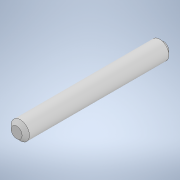
# Autodesk Inventor part: 3rd arm motor pin
Saved by Autodesk Inventor 2022 (Build 260153000, 153)
## iProperties
Created: 2021-07-07
Part Number: 3rd arm motor pin
Material: Generic
Document SubType Name: Modeling
Designer: USER
Density: 1 g/cm^3
Appearance: Default
Author: USER
Autodesk Inventor part; units mm, degrees
ref_plane "YZ Plane" through (0, 0, 0) normal (1, 0, 0) x (0, 1, 0)
ref_plane "XZ Plane" through (0, 0, 0) normal (0, 1, 0) x (-1, 0, 0)
ref_plane "XY Plane" through (0, 0, 0) normal (0, 0, 1) x (1, 0, 0)
sketch "Sketch1" plane through (0, 0, 0) normal (0, 0, 1) x (1, 0, 0)
  circle A0 centre (0, 0) radius 2.5
  dimension "d0" = 5
  constraints: 1 centre point, 1 coincident
  measures "d0" diameter of A0
extrude "Extrusion1" add sketch "Sketch1" along normal blind 40
chamfer "Chamfer1" distance 1 angle 45 2 edges at (-2.5, 0, 40) (-2.5, 0, 0)
body "Solid1"
